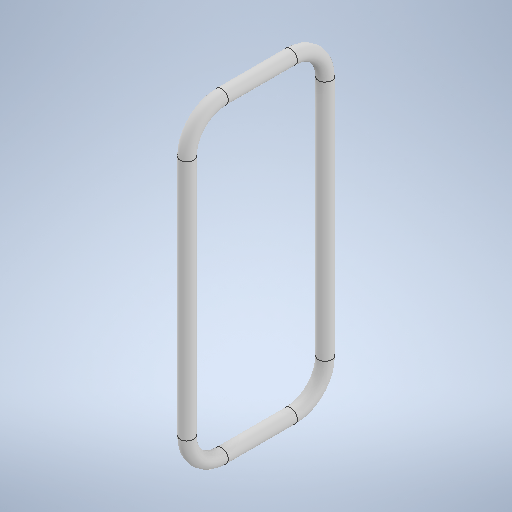
# Autodesk Inventor part: Mock String
Saved by Autodesk Inventor 2025.2 (Build 292293000, 293)
## iProperties
Created: 2025-02-17
Part Number: Mock String
Material: Generic
Document SubType Name: Modeling
Designer: baolo
Density: 1 g/cm^3
Appearance: Default
Author: baolo
Autodesk Inventor part; units mm, degrees
ref_plane "YZ Plane" through (0, 0, 0) normal (1, 0, 0) x (0, 1, 0)
ref_plane "XZ Plane" through (0, 0, 0) normal (0, 1, 0) x (-1, 0, 0)
ref_plane "XY Plane" through (0, 0, 0) normal (0, 0, 1) x (1, 0, 0)
sketch "Sketch1" plane through (0, 0, 0) normal (1, 0, 0) x (0, 1, 0)
  line L0 (17.5, 10) -> (-17.5, 10)
  line L1 (-22.5, 5) -> (-22.5, -5)
  line L2 (-17.5, -10) -> (17.5, -10)
  line L3 (22.5, -5) -> (22.5, 5)
  line L4 (22.5, 10) -> (-22.5, -10) construction
  line L5 (-22.5, 10) -> (22.5, -10) construction
  arc A0 (22.5, 5) -> (17.5, 10) centre (17.5, 5) ccw
  arc A1 (17.5, -10) -> (22.5, -5) centre (17.5, -5) ccw
  arc A2 (-22.5, -5) -> (-17.5, -10) centre (-17.5, -5) ccw
  arc A3 (-17.5, 10) -> (-22.5, 5) centre (-17.5, 5) ccw
  point P0 (0, 0)
  dimension "d0" = 45
  dimension "d1" = 20
  dimension "d2" = 5
  constraints: 12 end point, 8 point on circle, 8 point on line, 8 tangent, 4 centre point, 3 equal radius, 2 midpoint, 2 parallel, 1 horizontal, 1 perpendicular
  measures "d0" distance between parallel lines of L1 L3
  measures "d1" distance between parallel lines of L0 L2
  measures "d2" radius of A0
sketch "Sketch3" plane through (0, 0, 0) normal (0, 0, 1) x (1, 0, 0)
  circle A0 centre (0, 22.5) radius 1
  point P0 (0, 0)
  dimension "d4" = 2
  constraints: 1 centre point, 1 coincident
  measures "d4" diameter of A0
sweep "Sweep1" add profiles "Sketch3" path "Sketch1" path curves L3 A0 L0 A3 L1 A2 L2 A1
body "Solid1"
